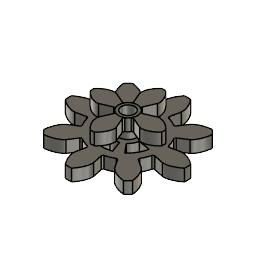
Gear 2 (Autodesk Fusion 360 design; units mm, degrees)
description: Spur Gear; Module: 12.700000; Num Teeth: 8; Pressure Angle: 20.000000; Backlash: 0.00 mm
description: Spur Gear; Module: 12.700000; Num Teeth: 4; Pressure Angle: 20.000000; Backlash: 0.00 mm
Autodesk Fusion 360 part; units mm, degrees
(part 1 of 2)
sketch "Sketch1" plane through (0, 0, 0) normal (0, 0, 1) x (1, 0, 0) in component "Spur Gear (8 teeth)"
  circle A0 centre (0, 0) radius 35.5092
  circle A1 centre (0, 0) radius 6.35
extrude "Extrude1" add sketch "Sketch1" along normal blind 12.7 makes body 1 in component "Spur Gear (8 teeth)"
sketch "Sketch2" plane through (0, 0, 0) normal (0, 0, 1) x (1, 0, 0) in component "Spur Gear (8 teeth)"
  spline S0 degree 5 poles (46.6751, -10.0097) (46.7226, -10.0198) (46.8178, -10.0383) (46.9612, -10.0605) (47.1537, -10.0796) (47.3962, -10.0893) (47.6398, -10.0891) (47.8842, -10.0829) (48.129, -10.0736) (48.374, -10.0619) (48.6191, -10.0476) (48.8645, -10.0296) (49.1102, -10.007) (49.3562, -9.9792) (49.6025, -9.9463) (49.849, -9.9089) (50.0955, -9.8676) (50.3422, -9.8231) (50.5887, -9.7758) (50.8353, -9.7255) (51.0817, -9.6724) (51.3281, -9.6161) (51.5744, -9.5567) (51.8206, -9.4939) (52.0667, -9.428) (52.3127, -9.3591) (52.5584, -9.2873) (52.804, -9.2128) (53.0494, -9.1355) (53.2944, -9.0557) (53.5393, -8.9732) (53.7839, -8.8881) (54.0281, -8.8003) (54.2721, -8.71) (54.5158, -8.617) (54.7591, -8.5215) (55.0021, -8.4236) (55.2447, -8.3232) (55.487, -8.2204) (55.7288, -8.1152) (55.9702, -8.0077) (56.2112, -7.8978) (56.4518, -7.7856) (56.6919, -7.6711) (56.9315, -7.5543) (57.1707, -7.4353) (57.4094, -7.314) (57.6476, -7.1905) (57.8853, -7.0648) (58.1224, -6.937) (58.3591, -6.807) (58.5951, -6.6749) (58.8307, -6.5406) (59.0656, -6.4043) (59.3, -6.2659) (59.5337, -6.1254) (59.7669, -5.9828) (59.9994, -5.8383) (60.2314, -5.6917) (60.4627, -5.5431) (60.6933, -5.3925) (60.9233, -5.24) (61.1526, -5.0855) (61.3813, -4.929) (61.6093, -4.7706) (61.8365, -4.6103) (62.0631, -4.4481) (62.2889, -4.2841) (62.5141, -4.1181) (62.7384, -3.9503) (62.9621, -3.7806) (63.1404, -3.6434) (63.2738, -3.5397) (63.3626, -3.4702) (63.407, -3.4353) knots 0 0 0 0 0 0 0.01428571 0.02857143 0.04285714 0.05714286 0.07142857 0.08571429 0.1 0.11428571 0.12857143 0.14285714 0.15714286 0.17142857 0.18571429 0.2 0.21428571 0.22857143 0.24285714 0.25714286 0.27142857 0.28571429 0.3 0.31428571 0.32857143 0.34285714 0.35714286 0.37142857 0.38571429 0.4 0.41428571 0.42857143 0.44285714 0.45714286 0.47142857 0.48571429 0.5 0.51428571 0.52857143 0.54285714 0.55714286 0.57142857 0.58571429 0.6 0.61428571 0.62857143 0.64285714 0.65714286 0.67142857 0.68571429 0.7 0.71428571 0.72857143 0.74285714 0.75714286 0.77142857 0.78571429 0.8 0.81428571 0.82857143 0.84285714 0.85714286 0.87142857 0.88571429 0.9 0.91428571 0.92857143 0.94285714 0.95714286 0.97142857 0.98571429 1 1 1 1 1 1
  spline S1 degree 5 poles (46.6751, 10.0097) (46.7226, 10.0198) (46.8178, 10.0383) (46.9612, 10.0605) (47.1537, 10.0796) (47.3962, 10.0893) (47.6398, 10.0891) (47.8842, 10.0829) (48.129, 10.0736) (48.374, 10.0619) (48.6191, 10.0476) (48.8645, 10.0296) (49.1102, 10.007) (49.3562, 9.9792) (49.6025, 9.9463) (49.849, 9.9089) (50.0955, 9.8676) (50.3422, 9.8231) (50.5887, 9.7758) (50.8353, 9.7255) (51.0817, 9.6724) (51.3281, 9.6161) (51.5744, 9.5567) (51.8206, 9.4939) (52.0667, 9.428) (52.3127, 9.3591) (52.5584, 9.2873) (52.804, 9.2128) (53.0494, 9.1355) (53.2944, 9.0557) (53.5393, 8.9732) (53.7839, 8.8881) (54.0281, 8.8003) (54.2721, 8.71) (54.5158, 8.617) (54.7591, 8.5215) (55.0021, 8.4236) (55.2447, 8.3232) (55.487, 8.2204) (55.7288, 8.1152) (55.9702, 8.0077) (56.2112, 7.8978) (56.4518, 7.7856) (56.6919, 7.6711) (56.9315, 7.5543) (57.1707, 7.4353) (57.4094, 7.314) (57.6476, 7.1905) (57.8853, 7.0648) (58.1224, 6.937) (58.3591, 6.807) (58.5951, 6.6749) (58.8307, 6.5406) (59.0656, 6.4043) (59.3, 6.2659) (59.5337, 6.1254) (59.7669, 5.9828) (59.9994, 5.8383) (60.2314, 5.6917) (60.4627, 5.5431) (60.6933, 5.3925) (60.9233, 5.24) (61.1526, 5.0855) (61.3813, 4.929) (61.6093, 4.7706) (61.8365, 4.6103) (62.0631, 4.4481) (62.2889, 4.2841) (62.5141, 4.1181) (62.7384, 3.9503) (62.9621, 3.7806) (63.1404, 3.6434) (63.2738, 3.5397) (63.3626, 3.4702) (63.407, 3.4353) knots 0 0 0 0 0 0 0.01428571 0.02857143 0.04285714 0.05714286 0.07142857 0.08571429 0.1 0.11428571 0.12857143 0.14285714 0.15714286 0.17142857 0.18571429 0.2 0.21428571 0.22857143 0.24285714 0.25714286 0.27142857 0.28571429 0.3 0.31428571 0.32857143 0.34285714 0.35714286 0.37142857 0.38571429 0.4 0.41428571 0.42857143 0.44285714 0.45714286 0.47142857 0.48571429 0.5 0.51428571 0.52857143 0.54285714 0.55714286 0.57142857 0.58571429 0.6 0.61428571 0.62857143 0.64285714 0.65714286 0.67142857 0.68571429 0.7 0.71428571 0.72857143 0.74285714 0.75714286 0.77142857 0.78571429 0.8 0.81428571 0.82857143 0.84285714 0.85714286 0.87142857 0.88571429 0.9 0.91428571 0.92857143 0.94285714 0.95714286 0.97142857 0.98571429 1 1 1 1 1 1
  arc A0 (63.407, -3.4353) -> (63.407, 3.4353) centre (0, 0) ccw
  line L0 (34.71, -7.4458) -> (46.6751, -10.0097)
  line L1 (34.71, 7.4458) -> (46.6751, 10.0097)
  line L2 (34.71, -7.4458) -> (34.71, 7.4458)
  point P0 (47.8104, -10.0842)
  point P1 (48.974, -10.0189)
  point P2 (50.155, -9.8564)
  point P3 (51.3487, -9.6105)
  point P4 (52.5517, -9.2886)
  point P5 (53.7613, -8.8954)
  point P6 (54.975, -8.434)
  point P7 (56.1906, -7.9067)
  point P8 (57.4059, -7.3152)
  point P9 (58.6189, -6.6609)
  point P10 (59.8275, -5.9448)
  point P11 (61.0296, -5.168)
  point P12 (62.2235, -4.3313)
  point P13 (47.8104, 10.0842)
  point P14 (48.974, 10.0189)
  point P15 (50.155, 9.8564)
  point P16 (51.3487, 9.6105)
  point P17 (52.5517, 9.2886)
  point P18 (53.7613, 8.8954)
  point P19 (54.975, 8.434)
  point P20 (56.1906, 7.9067)
  point P21 (57.4059, 7.3152)
  point P22 (58.6189, 6.6609)
  point P23 (59.8275, 5.9448)
  point P24 (61.0296, 5.168)
  point P25 (62.2235, 4.3313)
extrude "Extrude2" add sketch "Sketch2" along normal blind 12.7 bodies 1 in component "Spur Gear (8 teeth)"
fillet "Fillet1" radius 1.5875 2 edges at (34.7194, -7.4478, 6.35) (34.7194, 7.4478, 6.35) on bodies 1 in component "Spur Gear (8 teeth)"
pattern_circular "C-Pattern1" count 8 over 360 about axis through (0, 0, 0) along (0, 0, 1) of "Extrude2", "Fillet1" in component "Spur Gear (8 teeth)"
sketch "Sketch3" plane through (0, 0, 0) normal (0, 0, 1) x (1, 0, 0) in component "Spur Gear (8 teeth)"
  circle A0 centre (0, 0) radius 50.8 construction
sketch "Sketch1 (2)" plane through (0, 0, 0) normal (0, 0, 1) x (1, 0, 0) in component "Spur Gear (4 teeth)"
  circle A0 centre (0, 0) radius 10.1092
  circle A1 centre (0, 0) radius 6.35
extrude "Extrude1'" add sketch "Sketch1 (2)" along normal blind 12.7 separate body makes body 2 in component "Spur Gear (4 teeth)"
sketch "Sketch2 (2)" plane through (0, 0, 0) normal (0, 0, 1) x (1, 0, 0) in component "Spur Gear (4 teeth)"
  spline S0 degree 5 poles (21.9128, -9.4616) (21.9552, -9.4799) (22.0407, -9.5141) (22.1712, -9.5583) (22.3491, -9.6037) (22.5768, -9.6426) (22.8081, -9.6692) (23.0414, -9.6889) (23.2758, -9.7048) (23.5109, -9.7174) (23.7467, -9.7262) (23.9837, -9.7295) (24.2219, -9.7262) (24.4615, -9.7158) (24.7023, -9.6987) (24.9439, -9.6758) (25.1862, -9.648) (25.4288, -9.6159) (25.6717, -9.5798) (25.9149, -9.5397) (26.1582, -9.4952) (26.4018, -9.4462) (26.6456, -9.3926) (26.8896, -9.3344) (27.1337, -9.2719) (27.3777, -9.2051) (27.6217, -9.1343) (27.8655, -9.0596) (28.109, -8.9811) (28.3523, -8.8987) (28.5954, -8.8125) (28.838, -8.7225) (29.0803, -8.6286) (29.3222, -8.531) (29.5637, -8.4296) (29.8046, -8.3246) (30.045, -8.216) (30.2848, -8.1038) (30.5239, -7.9882) (30.7623, -7.869) (31.0001, -7.7465) (31.2371, -7.6205) (31.4733, -7.491) (31.7087, -7.3583) (31.9432, -7.2221) (32.1769, -7.0827) (32.4096, -6.9401) (32.6414, -6.7942) (32.8722, -6.6451) (33.1019, -6.4928) (33.3306, -6.3374) (33.5583, -6.1789) (33.7848, -6.0173) (34.0102, -5.8526) (34.2343, -5.6849) (34.4573, -5.5142) (34.6791, -5.3405) (34.8996, -5.1639) (35.1188, -4.9843) (35.3367, -4.8018) (35.5532, -4.6165) (35.7684, -4.4283) (35.9823, -4.2373) (36.1947, -4.0436) (36.4056, -3.847) (36.6151, -3.6477) (36.823, -3.4457) (37.0294, -3.241) (37.2343, -3.0337) (37.4376, -2.8237) (37.6393, -2.6111) (37.7995, -2.4389) (37.9189, -2.3086) (37.9982, -2.2212) (38.0377, -2.1774) knots 0 0 0 0 0 0 0.01428571 0.02857143 0.04285714 0.05714286 0.07142857 0.08571429 0.1 0.11428571 0.12857143 0.14285714 0.15714286 0.17142857 0.18571429 0.2 0.21428571 0.22857143 0.24285714 0.25714286 0.27142857 0.28571429 0.3 0.31428571 0.32857143 0.34285714 0.35714286 0.37142857 0.38571429 0.4 0.41428571 0.42857143 0.44285714 0.45714286 0.47142857 0.48571429 0.5 0.51428571 0.52857143 0.54285714 0.55714286 0.57142857 0.58571429 0.6 0.61428571 0.62857143 0.64285714 0.65714286 0.67142857 0.68571429 0.7 0.71428571 0.72857143 0.74285714 0.75714286 0.77142857 0.78571429 0.8 0.81428571 0.82857143 0.84285714 0.85714286 0.87142857 0.88571429 0.9 0.91428571 0.92857143 0.94285714 0.95714286 0.97142857 0.98571429 1 1 1 1 1 1
  spline S1 degree 5 poles (21.9128, 9.4616) (21.9552, 9.4799) (22.0407, 9.5141) (22.1712, 9.5583) (22.3491, 9.6037) (22.5768, 9.6426) (22.8081, 9.6692) (23.0414, 9.6889) (23.2758, 9.7048) (23.5109, 9.7174) (23.7467, 9.7262) (23.9837, 9.7295) (24.2219, 9.7262) (24.4615, 9.7158) (24.7023, 9.6987) (24.9439, 9.6758) (25.1862, 9.648) (25.4288, 9.6159) (25.6717, 9.5798) (25.9149, 9.5397) (26.1582, 9.4952) (26.4018, 9.4462) (26.6456, 9.3926) (26.8896, 9.3344) (27.1337, 9.2719) (27.3777, 9.2051) (27.6217, 9.1343) (27.8655, 9.0596) (28.109, 8.9811) (28.3523, 8.8987) (28.5954, 8.8125) (28.838, 8.7225) (29.0803, 8.6286) (29.3222, 8.531) (29.5637, 8.4296) (29.8046, 8.3246) (30.045, 8.216) (30.2848, 8.1038) (30.5239, 7.9882) (30.7623, 7.869) (31.0001, 7.7465) (31.2371, 7.6205) (31.4733, 7.491) (31.7087, 7.3583) (31.9432, 7.2221) (32.1769, 7.0827) (32.4096, 6.9401) (32.6414, 6.7942) (32.8722, 6.6451) (33.1019, 6.4928) (33.3306, 6.3374) (33.5583, 6.1789) (33.7848, 6.0173) (34.0102, 5.8526) (34.2343, 5.6849) (34.4573, 5.5142) (34.6791, 5.3405) (34.8996, 5.1639) (35.1188, 4.9843) (35.3367, 4.8018) (35.5532, 4.6165) (35.7684, 4.4283) (35.9823, 4.2373) (36.1947, 4.0436) (36.4056, 3.847) (36.6151, 3.6477) (36.823, 3.4457) (37.0294, 3.241) (37.2343, 3.0337) (37.4376, 2.8237) (37.6393, 2.6111) (37.7995, 2.4389) (37.9189, 2.3086) (37.9982, 2.2212) (38.0377, 2.1774) knots 0 0 0 0 0 0 0.01428571 0.02857143 0.04285714 0.05714286 0.07142857 0.08571429 0.1 0.11428571 0.12857143 0.14285714 0.15714286 0.17142857 0.18571429 0.2 0.21428571 0.22857143 0.24285714 0.25714286 0.27142857 0.28571429 0.3 0.31428571 0.32857143 0.34285714 0.35714286 0.37142857 0.38571429 0.4 0.41428571 0.42857143 0.44285714 0.45714286 0.47142857 0.48571429 0.5 0.51428571 0.52857143 0.54285714 0.55714286 0.57142857 0.58571429 0.6 0.61428571 0.62857143 0.64285714 0.65714286 0.67142857 0.68571429 0.7 0.71428571 0.72857143 0.74285714 0.75714286 0.77142857 0.78571429 0.8 0.81428571 0.82857143 0.84285714 0.85714286 0.87142857 0.88571429 0.9 0.91428571 0.92857143 0.94285714 0.95714286 0.97142857 0.98571429 1 1 1 1 1 1
  arc A0 (38.0377, -2.1774) -> (38.0377, 2.1774) centre (0, 0) ccw
  line L0 (9.2718, -4.0074) -> (21.9128, -9.4616)
  line L1 (9.2718, 4.0074) -> (21.9128, 9.4616)
  line L2 (9.2718, -4.0074) -> (9.2718, 4.0074)
  point P0 (22.9255, -9.6784)
  point P1 (24.0052, -9.7278)
  point P2 (25.1271, -9.6541)
  point P3 (26.2802, -9.4701)
  point P4 (27.4564, -9.1817)
  point P5 (28.6488, -8.792)
  point P6 (29.8509, -8.303)
  point P7 (31.0565, -7.7159)
  point P8 (32.2598, -7.0314)
  point P9 (33.4549, -6.2504)
  point P10 (34.636, -5.3736)
  point P11 (35.7973, -4.4018)
  point P12 (36.9331, -3.336)
  point P13 (22.9255, 9.6784)
  point P14 (24.0052, 9.7278)
  point P15 (25.1271, 9.6541)
  point P16 (26.2802, 9.4701)
  point P17 (27.4564, 9.1817)
  point P18 (28.6488, 8.792)
  point P19 (29.8509, 8.303)
  point P20 (31.0565, 7.7159)
  point P21 (32.2598, 7.0314)
  point P22 (33.4549, 6.2504)
  point P23 (34.636, 5.3736)
  point P24 (35.7973, 4.4018)
  point P25 (36.9331, 3.336)
extrude "Extrude2'" add sketch "Sketch2 (2)" along normal blind 12.7 bodies 2 in component "Spur Gear (4 teeth)"
fillet "Fillet1'" radius 1.5875 2 edges at (9.2795, -4.0107, 6.35) (9.2795, 4.0107, 6.35) on bodies 2 in component "Spur Gear (4 teeth)"
pattern_circular "C-Pattern1'" count 4 over 360 about axis through (0, 0, 0) along (0, 0, 1) of "Extrude2'", "Fillet1'" in component "Spur Gear (4 teeth)"
sketch "Sketch3 (2)" plane through (0, 0, 0) normal (0, 0, 1) x (1, 0, 0) in component "Spur Gear (4 teeth)"
  circle A0 centre (0, 0) radius 25.4 construction
move_body "Move1" bodies 2 to x (1, 0, 0) y (0, 1, 0) z (0, 0, 1) at (0, 0, 20) in component "Spur Gear (4 teeth)"
sketch "Sketch1 (3)" plane through (0, 0, 0) normal (0, 0, -1) x (1, 0, 0)
  circle A0 centre (0, 0) radius 6.35
  arc A1 (7.7732, 36.2381) -> (8.9264, 34.3689) centre (9.3255, 35.9054) ccw
  line L0 (7.7732, 36.2381) -> (10.0097, 46.6751)
  spline S0 degree 5 poles (10.0097, 46.6751) (10.0198, 46.7226) (10.0383, 46.8178) (10.0605, 46.9612) (10.0796, 47.1537) (10.0893, 47.3962) (10.0891, 47.6398) (10.0829, 47.8842) (10.0736, 48.129) (10.0619, 48.374) (10.0476, 48.6191) (10.0296, 48.8645) (10.007, 49.1102) (9.9792, 49.3562) (9.9463, 49.6025) (9.9089, 49.849) (9.8676, 50.0955) (9.8231, 50.3422) (9.7758, 50.5887) (9.7255, 50.8353) (9.6724, 51.0817) (9.6161, 51.3281) (9.5567, 51.5744) (9.4939, 51.8206) (9.428, 52.0667) (9.3591, 52.3127) (9.2873, 52.5584) (9.2128, 52.804) (9.1355, 53.0494) (9.0557, 53.2944) (8.9732, 53.5393) (8.8881, 53.7839) (8.8003, 54.0281) (8.71, 54.2721) (8.617, 54.5158) (8.5215, 54.7591) (8.4236, 55.0021) (8.3232, 55.2447) (8.2204, 55.487) (8.1152, 55.7288) (8.0077, 55.9702) (7.8978, 56.2112) (7.7856, 56.4518) (7.6711, 56.6919) (7.5543, 56.9315) (7.4353, 57.1707) (7.314, 57.4094) (7.1905, 57.6476) (7.0648, 57.8853) (6.937, 58.1224) (6.807, 58.3591) (6.6749, 58.5951) (6.5406, 58.8307) (6.4043, 59.0656) (6.2659, 59.3) (6.1254, 59.5337) (5.9828, 59.7669) (5.8383, 59.9994) (5.6917, 60.2314) (5.5431, 60.4627) (5.3925, 60.6933) (5.24, 60.9233) (5.0855, 61.1526) (4.929, 61.3813) (4.7706, 61.6093) (4.6103, 61.8365) (4.4481, 62.0631) (4.2841, 62.2889) (4.1181, 62.5141) (3.9503, 62.7384) (3.7806, 62.9621) (3.6434, 63.1404) (3.5397, 63.2738) (3.4702, 63.3626) (3.4353, 63.407) knots 0 0 0 0 0 0 0.01428571 0.02857143 0.04285714 0.05714286 0.07142857 0.08571429 0.1 0.11428571 0.12857143 0.14285714 0.15714286 0.17142857 0.18571429 0.2 0.21428571 0.22857143 0.24285714 0.25714286 0.27142857 0.28571429 0.3 0.31428571 0.32857143 0.34285714 0.35714286 0.37142857 0.38571429 0.4 0.41428571 0.42857143 0.44285714 0.45714286 0.47142857 0.48571429 0.5 0.51428571 0.52857143 0.54285714 0.55714286 0.57142857 0.58571429 0.6 0.61428571 0.62857143 0.64285714 0.65714286 0.67142857 0.68571429 0.7 0.71428571 0.72857143 0.74285714 0.75714286 0.77142857 0.78571429 0.8 0.81428571 0.82857143 0.84285714 0.85714286 0.87142857 0.88571429 0.9 0.91428571 0.92857143 0.94285714 0.95714286 0.97142857 0.98571429 1 1 1 1 1 1
  arc A2 (3.4353, 63.407) -> (-3.4353, 63.407) centre (0, 0) ccw
  spline S1 degree 5 poles (-10.0097, 46.6751) (-10.0198, 46.7226) (-10.0383, 46.8178) (-10.0605, 46.9612) (-10.0796, 47.1537) (-10.0893, 47.3962) (-10.0891, 47.6398) (-10.0829, 47.8842) (-10.0736, 48.129) (-10.0619, 48.374) (-10.0476, 48.6191) (-10.0296, 48.8645) (-10.007, 49.1102) (-9.9792, 49.3562) (-9.9463, 49.6025) (-9.9089, 49.849) (-9.8676, 50.0955) (-9.8231, 50.3422) (-9.7758, 50.5887) (-9.7255, 50.8353) (-9.6724, 51.0817) (-9.6161, 51.3281) (-9.5567, 51.5744) (-9.4939, 51.8206) (-9.428, 52.0667) (-9.3591, 52.3127) (-9.2873, 52.5584) (-9.2128, 52.804) (-9.1355, 53.0494) (-9.0557, 53.2944) (-8.9732, 53.5393) (-8.8881, 53.7839) (-8.8003, 54.0281) (-8.71, 54.2721) (-8.617, 54.5158) (-8.5215, 54.7591) (-8.4236, 55.0021) (-8.3232, 55.2447) (-8.2204, 55.487) (-8.1152, 55.7288) (-8.0077, 55.9702) (-7.8978, 56.2112) (-7.7856, 56.4518) (-7.6711, 56.6919) (-7.5543, 56.9315) (-7.4353, 57.1707) (-7.314, 57.4094) (-7.1905, 57.6476) (-7.0648, 57.8853) (-6.937, 58.1224) (-6.807, 58.3591) (-6.6749, 58.5951) (-6.5406, 58.8307) (-6.4043, 59.0656) (-6.2659, 59.3) (-6.1254, 59.5337) (-5.9828, 59.7669) (-5.8383, 59.9994) (-5.6917, 60.2314) (-5.5431, 60.4627) (-5.3925, 60.6933) (-5.24, 60.9233) (-5.0855, 61.1526) (-4.929, 61.3813) (-4.7706, 61.6093) (-4.6103, 61.8365) (-4.4481, 62.0631) (-4.2841, 62.2889) (-4.1181, 62.5141) (-3.9503, 62.7384) (-3.7806, 62.9621) (-3.6434, 63.1404) (-3.5397, 63.2738) (-3.4702, 63.3626) (-3.4353, 63.407) knots 0 0 0 0 0 0 0.01428571 0.02857143 0.04285714 0.05714286 0.07142857 0.08571429 0.1 0.11428571 0.12857143 0.14285714 0.15714286 0.17142857 0.18571429 0.2 0.21428571 0.22857143 0.24285714 0.25714286 0.27142857 0.28571429 0.3 0.31428571 0.32857143 0.34285714 0.35714286 0.37142857 0.38571429 0.4 0.41428571 0.42857143 0.44285714 0.45714286 0.47142857 0.48571429 0.5 0.51428571 0.52857143 0.54285714 0.55714286 0.57142857 0.58571429 0.6 0.61428571 0.62857143 0.64285714 0.65714286 0.67142857 0.68571429 0.7 0.71428571 0.72857143 0.74285714 0.75714286 0.77142857 0.78571429 0.8 0.81428571 0.82857143 0.84285714 0.85714286 0.87142857 0.88571429 0.9 0.91428571 0.92857143 0.94285714 0.95714286 0.97142857 0.98571429 1 1 1 1 1 1
  line L1 (-10.0097, 46.6751) -> (-7.7732, 36.2381)
  arc A3 (-8.9264, 34.3689) -> (-7.7732, 36.2381) centre (-9.3255, 35.9054) ccw
  arc A4 (-8.9264, 34.3689) -> (-17.9906, 30.6144) centre (0, 0) ccw
  arc A5 (-20.1277, 31.1207) -> (-17.9906, 30.6144) centre (-18.7949, 31.9831) ccw
  line L2 (-20.1277, 31.1207) -> (-25.9264, 40.0822)
  spline S2 degree 5 poles (-25.9264, 40.0822) (-25.9528, 40.123) (-26.007, 40.2033) (-26.0927, 40.3204) (-26.2154, 40.4701) (-26.3799, 40.6484) (-26.5524, 40.8205) (-26.7296, 40.989) (-26.9092, 41.1554) (-27.0907, 41.3204) (-27.2742, 41.4836) (-27.4604, 41.6444) (-27.6501, 41.8022) (-27.8437, 41.9565) (-28.0411, 42.1074) (-28.2419, 42.2552) (-28.4454, 42.4004) (-28.6513, 42.5433) (-28.8591, 42.6841) (-29.069, 42.823) (-29.2808, 42.9596) (-29.4948, 43.0941) (-29.711, 43.2262) (-29.9295, 43.3559) (-30.1501, 43.4833) (-30.3728, 43.6085) (-30.5973, 43.7315) (-30.8237, 43.8525) (-31.0517, 43.9714) (-31.2815, 44.0882) (-31.513, 44.203) (-31.7461, 44.3158) (-31.9809, 44.4264) (-32.2173, 44.5351) (-32.4553, 44.6416) (-32.6949, 44.7462) (-32.936, 44.8487) (-33.1785, 44.9493) (-33.4225, 45.0479) (-33.6679, 45.1445) (-33.9146, 45.2392) (-34.1627, 45.3319) (-34.4122, 45.4227) (-34.6629, 45.5115) (-34.915, 45.5984) (-35.1683, 45.6833) (-35.4228, 45.7664) (-35.6786, 45.8475) (-35.9355, 45.9267) (-36.1936, 46.004) (-36.4528, 46.0794) (-36.7132, 46.1529) (-36.9746, 46.2245) (-37.2372, 46.2942) (-37.5008, 46.362) (-37.7654, 46.428) (-38.0311, 46.4921) (-38.2977, 46.5543) (-38.5654, 46.6146) (-38.834, 46.6731) (-39.1036, 46.7297) (-39.3741, 46.7845) (-39.6455, 46.8374) (-39.9178, 46.8885) (-40.191, 46.9377) (-40.465, 46.985) (-40.7399, 47.0305) (-41.0156, 47.0742) (-41.2922, 47.1161) (-41.5695, 47.1561) (-41.8476, 47.1942) (-42.0707, 47.2233) (-42.2384, 47.2443) (-42.3504, 47.2579) (-42.4064, 47.2647) knots 0 0 0 0 0 0 0.01428571 0.02857143 0.04285714 0.05714286 0.07142857 0.08571429 0.1 0.11428571 0.12857143 0.14285714 0.15714286 0.17142857 0.18571429 0.2 0.21428571 0.22857143 0.24285714 0.25714286 0.27142857 0.28571429 0.3 0.31428571 0.32857143 0.34285714 0.35714286 0.37142857 0.38571429 0.4 0.41428571 0.42857143 0.44285714 0.45714286 0.47142857 0.48571429 0.5 0.51428571 0.52857143 0.54285714 0.55714286 0.57142857 0.58571429 0.6 0.61428571 0.62857143 0.64285714 0.65714286 0.67142857 0.68571429 0.7 0.71428571 0.72857143 0.74285714 0.75714286 0.77142857 0.78571429 0.8 0.81428571 0.82857143 0.84285714 0.85714286 0.87142857 0.88571429 0.9 0.91428571 0.92857143 0.94285714 0.95714286 0.97142857 0.98571429 1 1 1 1 1 1
  arc A6 (-42.4064, 47.2647) -> (-47.2647, 42.4064) centre (0, 0) ccw
  spline S3 degree 5 poles (-40.0822, 25.9264) (-40.123, 25.9528) (-40.2033, 26.007) (-40.3204, 26.0927) (-40.4701, 26.2154) (-40.6484, 26.3799) (-40.8205, 26.5524) (-40.989, 26.7296) (-41.1554, 26.9092) (-41.3204, 27.0907) (-41.4836, 27.2742) (-41.6444, 27.4604) (-41.8022, 27.6501) (-41.9565, 27.8437) (-42.1074, 28.0411) (-42.2552, 28.2419) (-42.4004, 28.4454) (-42.5433, 28.6513) (-42.6841, 28.8591) (-42.823, 29.069) (-42.9596, 29.2808) (-43.0941, 29.4948) (-43.2262, 29.711) (-43.3559, 29.9295) (-43.4833, 30.1501) (-43.6085, 30.3728) (-43.7315, 30.5973) (-43.8525, 30.8237) (-43.9714, 31.0517) (-44.0882, 31.2815) (-44.203, 31.513) (-44.3158, 31.7461) (-44.4264, 31.9809) (-44.5351, 32.2173) (-44.6416, 32.4553) (-44.7462, 32.6949) (-44.8487, 32.936) (-44.9493, 33.1785) (-45.0479, 33.4225) (-45.1445, 33.6679) (-45.2392, 33.9146) (-45.3319, 34.1627) (-45.4227, 34.4122) (-45.5115, 34.6629) (-45.5984, 34.915) (-45.6833, 35.1683) (-45.7664, 35.4228) (-45.8475, 35.6786) (-45.9267, 35.9355) (-46.004, 36.1936) (-46.0794, 36.4528) (-46.1529, 36.7132) (-46.2245, 36.9746) (-46.2942, 37.2372) (-46.362, 37.5008) (-46.428, 37.7654) (-46.4921, 38.0311) (-46.5543, 38.2977) (-46.6146, 38.5654) (-46.6731, 38.834) (-46.7297, 39.1036) (-46.7845, 39.3741) (-46.8374, 39.6455) (-46.8885, 39.9178) (-46.9377, 40.191) (-46.985, 40.465) (-47.0305, 40.7399) (-47.0742, 41.0156) (-47.1161, 41.2922) (-47.1561, 41.5695) (-47.1942, 41.8476) (-47.2233, 42.0707) (-47.2443, 42.2384) (-47.2579, 42.3504) (-47.2647, 42.4064) knots 0 0 0 0 0 0 0.01428571 0.02857143 0.04285714 0.05714286 0.07142857 0.08571429 0.1 0.11428571 0.12857143 0.14285714 0.15714286 0.17142857 0.18571429 0.2 0.21428571 0.22857143 0.24285714 0.25714286 0.27142857 0.28571429 0.3 0.31428571 0.32857143 0.34285714 0.35714286 0.37142857 0.38571429 0.4 0.41428571 0.42857143 0.44285714 0.45714286 0.47142857 0.48571429 0.5 0.51428571 0.52857143 0.54285714 0.55714286 0.57142857 0.58571429 0.6 0.61428571 0.62857143 0.64285714 0.65714286 0.67142857 0.68571429 0.7 0.71428571 0.72857143 0.74285714 0.75714286 0.77142857 0.78571429 0.8 0.81428571 0.82857143 0.84285714 0.85714286 0.87142857 0.88571429 0.9 0.91428571 0.92857143 0.94285714 0.95714286 0.97142857 0.98571429 1 1 1 1 1 1
  line L3 (-40.0822, 25.9264) -> (-31.1207, 20.1277)
  arc A7 (-30.6144, 17.9906) -> (-31.1207, 20.1277) centre (-31.9831, 18.7949) ccw
  arc A8 (-30.6144, 17.9906) -> (-34.3689, 8.9264) centre (0, 0) ccw
  arc A9 (-36.2381, 7.7732) -> (-34.3689, 8.9264) centre (-35.9054, 9.3255) ccw
  line L4 (-36.2381, 7.7732) -> (-46.6751, 10.0097)
  spline S4 degree 5 poles (-46.6751, 10.0097) (-46.7226, 10.0198) (-46.8178, 10.0383) (-46.9612, 10.0605) (-47.1537, 10.0796) (-47.3962, 10.0893) (-47.6398, 10.0891) (-47.8842, 10.0829) (-48.129, 10.0736) (-48.374, 10.0619) (-48.6191, 10.0476) (-48.8645, 10.0296) (-49.1102, 10.007) (-49.3562, 9.9792) (-49.6025, 9.9463) (-49.849, 9.9089) (-50.0955, 9.8676) (-50.3422, 9.8231) (-50.5887, 9.7758) (-50.8353, 9.7255) (-51.0817, 9.6724) (-51.3281, 9.6161) (-51.5744, 9.5567) (-51.8206, 9.4939) (-52.0667, 9.428) (-52.3127, 9.3591) (-52.5584, 9.2873) (-52.804, 9.2128) (-53.0494, 9.1355) (-53.2944, 9.0557) (-53.5393, 8.9732) (-53.7839, 8.8881) (-54.0281, 8.8003) (-54.2721, 8.71) (-54.5158, 8.617) (-54.7591, 8.5215) (-55.0021, 8.4236) (-55.2447, 8.3232) (-55.487, 8.2204) (-55.7288, 8.1152) (-55.9702, 8.0077) (-56.2112, 7.8978) (-56.4518, 7.7856) (-56.6919, 7.6711) (-56.9315, 7.5543) (-57.1707, 7.4353) (-57.4094, 7.314) (-57.6476, 7.1905) (-57.8853, 7.0648) (-58.1224, 6.937) (-58.3591, 6.807) (-58.5951, 6.6749) (-58.8307, 6.5406) (-59.0656, 6.4043) (-59.3, 6.2659) (-59.5337, 6.1254) (-59.7669, 5.9828) (-59.9994, 5.8383) (-60.2314, 5.6917) (-60.4627, 5.5431) (-60.6933, 5.3925) (-60.9233, 5.24) (-61.1526, 5.0855) (-61.3813, 4.929) (-61.6093, 4.7706) (-61.8365, 4.6103) (-62.0631, 4.4481) (-62.2889, 4.2841) (-62.5141, 4.1181) (-62.7384, 3.9503) (-62.9621, 3.7806) (-63.1404, 3.6434) (-63.2738, 3.5397) (-63.3626, 3.4702) (-63.407, 3.4353) knots 0 0 0 0 0 0 0.01428571 0.02857143 0.04285714 0.05714286 0.07142857 0.08571429 0.1 0.11428571 0.12857143 0.14285714 0.15714286 0.17142857 0.18571429 0.2 0.21428571 0.22857143 0.24285714 0.25714286 0.27142857 0.28571429 0.3 0.31428571 0.32857143 0.34285714 0.35714286 0.37142857 0.38571429 0.4 0.41428571 0.42857143 0.44285714 0.45714286 0.47142857 0.48571429 0.5 0.51428571 0.52857143 0.54285714 0.55714286 0.57142857 0.58571429 0.6 0.61428571 0.62857143 0.64285714 0.65714286 0.67142857 0.68571429 0.7 0.71428571 0.72857143 0.74285714 0.75714286 0.77142857 0.78571429 0.8 0.81428571 0.82857143 0.84285714 0.85714286 0.87142857 0.88571429 0.9 0.91428571 0.92857143 0.94285714 0.95714286 0.97142857 0.98571429 1 1 1 1 1 1
  arc A10 (-63.407, 3.4353) -> (-63.407, -3.4353) centre (0, 0) ccw
  spline S5 degree 5 poles (-46.6751, -10.0097) (-46.7226, -10.0198) (-46.8178, -10.0383) (-46.9612, -10.0605) (-47.1537, -10.0796) (-47.3962, -10.0893) (-47.6398, -10.0891) (-47.8842, -10.0829) (-48.129, -10.0736) (-48.374, -10.0619) (-48.6191, -10.0476) (-48.8645, -10.0296) (-49.1102, -10.007) (-49.3562, -9.9792) (-49.6025, -9.9463) (-49.849, -9.9089) (-50.0955, -9.8676) (-50.3422, -9.8231) (-50.5887, -9.7758) (-50.8353, -9.7255) (-51.0817, -9.6724) (-51.3281, -9.6161) (-51.5744, -9.5567) (-51.8206, -9.4939) (-52.0667, -9.428) (-52.3127, -9.3591) (-52.5584, -9.2873) (-52.804, -9.2128) (-53.0494, -9.1355) (-53.2944, -9.0557) (-53.5393, -8.9732) (-53.7839, -8.8881) (-54.0281, -8.8003) (-54.2721, -8.71) (-54.5158, -8.617) (-54.7591, -8.5215) (-55.0021, -8.4236) (-55.2447, -8.3232) (-55.487, -8.2204) (-55.7288, -8.1152) (-55.9702, -8.0077) (-56.2112, -7.8978) (-56.4518, -7.7856) (-56.6919, -7.6711) (-56.9315, -7.5543) (-57.1707, -7.4353) (-57.4094, -7.314) (-57.6476, -7.1905) (-57.8853, -7.0648) (-58.1224, -6.937) (-58.3591, -6.807) (-58.5951, -6.6749) (-58.8307, -6.5406) (-59.0656, -6.4043) (-59.3, -6.2659) (-59.5337, -6.1254) (-59.7669, -5.9828) (-59.9994, -5.8383) (-60.2314, -5.6917) (-60.4627, -5.5431) (-60.6933, -5.3925) (-60.9233, -5.24) (-61.1526, -5.0855) (-61.3813, -4.929) (-61.6093, -4.7706) (-61.8365, -4.6103) (-62.0631, -4.4481) (-62.2889, -4.2841) (-62.5141, -4.1181) (-62.7384, -3.9503) (-62.9621, -3.7806) (-63.1404, -3.6434) (-63.2738, -3.5397) (-63.3626, -3.4702) (-63.407, -3.4353) knots 0 0 0 0 0 0 0.01428571 0.02857143 0.04285714 0.05714286 0.07142857 0.08571429 0.1 0.11428571 0.12857143 0.14285714 0.15714286 0.17142857 0.18571429 0.2 0.21428571 0.22857143 0.24285714 0.25714286 0.27142857 0.28571429 0.3 0.31428571 0.32857143 0.34285714 0.35714286 0.37142857 0.38571429 0.4 0.41428571 0.42857143 0.44285714 0.45714286 0.47142857 0.48571429 0.5 0.51428571 0.52857143 0.54285714 0.55714286 0.57142857 0.58571429 0.6 0.61428571 0.62857143 0.64285714 0.65714286 0.67142857 0.68571429 0.7 0.71428571 0.72857143 0.74285714 0.75714286 0.77142857 0.78571429 0.8 0.81428571 0.82857143 0.84285714 0.85714286 0.87142857 0.88571429 0.9 0.91428571 0.92857143 0.94285714 0.95714286 0.97142857 0.98571429 1 1 1 1 1 1
  line L5 (-46.6751, -10.0097) -> (-36.2381, -7.7732)
  arc A11 (-34.3689, -8.9264) -> (-36.2381, -7.7732) centre (-35.9054, -9.3255) ccw
  arc A12 (-34.3689, -8.9264) -> (-30.6144, -17.9906) centre (0, 0) ccw
  arc A13 (-31.1207, -20.1277) -> (-30.6144, -17.9906) centre (-31.9831, -18.7949) ccw
  line L6 (-31.1207, -20.1277) -> (-40.0822, -25.9264)
  spline S6 degree 5 poles (-40.0822, -25.9264) (-40.123, -25.9528) (-40.2033, -26.007) (-40.3204, -26.0927) (-40.4701, -26.2154) (-40.6484, -26.3799) (-40.8205, -26.5524) (-40.989, -26.7296) (-41.1554, -26.9092) (-41.3204, -27.0907) (-41.4836, -27.2742) (-41.6444, -27.4604) (-41.8022, -27.6501) (-41.9565, -27.8437) (-42.1074, -28.0411) (-42.2552, -28.2419) (-42.4004, -28.4454) (-42.5433, -28.6513) (-42.6841, -28.8591) (-42.823, -29.069) (-42.9596, -29.2808) (-43.0941, -29.4948) (-43.2262, -29.711) (-43.3559, -29.9295) (-43.4833, -30.1501) (-43.6085, -30.3728) (-43.7315, -30.5973) (-43.8525, -30.8237) (-43.9714, -31.0517) (-44.0882, -31.2815) (-44.203, -31.513) (-44.3158, -31.7461) (-44.4264, -31.9809) (-44.5351, -32.2173) (-44.6416, -32.4553) (-44.7462, -32.6949) (-44.8487, -32.936) (-44.9493, -33.1785) (-45.0479, -33.4225) (-45.1445, -33.6679) (-45.2392, -33.9146) (-45.3319, -34.1627) (-45.4227, -34.4122) (-45.5115, -34.6629) (-45.5984, -34.915) (-45.6833, -35.1683) (-45.7664, -35.4228) (-45.8475, -35.6786) (-45.9267, -35.9355) (-46.004, -36.1936) (-46.0794, -36.4528) (-46.1529, -36.7132) (-46.2245, -36.9746) (-46.2942, -37.2372) (-46.362, -37.5008) (-46.428, -37.7654) (-46.4921, -38.0311) (-46.5543, -38.2977) (-46.6146, -38.5654) (-46.6731, -38.834) (-46.7297, -39.1036) (-46.7845, -39.3741) (-46.8374, -39.6455) (-46.8885, -39.9178) (-46.9377, -40.191) (-46.985, -40.465) (-47.0305, -40.7399) (-47.0742, -41.0156) (-47.1161, -41.2922) (-47.1561, -41.5695) (-47.1942, -41.8476) (-47.2233, -42.0707) (-47.2443, -42.2384) (-47.2579, -42.3504) (-47.2647, -42.4064) knots 0 0 0 0 0 0 0.01428571 0.02857143 0.04285714 0.05714286 0.07142857 0.08571429 0.1 0.11428571 0.12857143 0.14285714 0.15714286 0.17142857 0.18571429 0.2 0.21428571 0.22857143 0.24285714 0.25714286 0.27142857 0.28571429 0.3 0.31428571 0.32857143 0.34285714 0.35714286 0.37142857 0.38571429 0.4 0.41428571 0.42857143 0.44285714 0.45714286 0.47142857 0.48571429 0.5 0.51428571 0.52857143 0.54285714 0.55714286 0.57142857 0.58571429 0.6 0.61428571 0.62857143 0.64285714 0.65714286 0.67142857 0.68571429 0.7 0.71428571 0.72857143 0.74285714 0.75714286 0.77142857 0.78571429 0.8 0.81428571 0.82857143 0.84285714 0.85714286 0.87142857 0.88571429 0.9 0.91428571 0.92857143 0.94285714 0.95714286 0.97142857 0.98571429 1 1 1 1 1 1
  arc A14 (-47.2647, -42.4064) -> (-42.4064, -47.2647) centre (0, 0) ccw
  spline S7 degree 5 poles (-25.9264, -40.0822) (-25.9528, -40.123) (-26.007, -40.2033) (-26.0927, -40.3204) (-26.2154, -40.4701) (-26.3799, -40.6484) (-26.5524, -40.8205) (-26.7296, -40.989) (-26.9092, -41.1554) (-27.0907, -41.3204) (-27.2742, -41.4836) (-27.4604, -41.6444) (-27.6501, -41.8022) (-27.8437, -41.9565) (-28.0411, -42.1074) (-28.2419, -42.2552) (-28.4454, -42.4004) (-28.6513, -42.5433) (-28.8591, -42.6841) (-29.069, -42.823) (-29.2808, -42.9596) (-29.4948, -43.0941) (-29.711, -43.2262) (-29.9295, -43.3559) (-30.1501, -43.4833) (-30.3728, -43.6085) (-30.5973, -43.7315) (-30.8237, -43.8525) (-31.0517, -43.9714) (-31.2815, -44.0882) (-31.513, -44.203) (-31.7461, -44.3158) (-31.9809, -44.4264) (-32.2173, -44.5351) (-32.4553, -44.6416) (-32.6949, -44.7462) (-32.936, -44.8487) (-33.1785, -44.9493) (-33.4225, -45.0479) (-33.6679, -45.1445) (-33.9146, -45.2392) (-34.1627, -45.3319) (-34.4122, -45.4227) (-34.6629, -45.5115) (-34.915, -45.5984) (-35.1683, -45.6833) (-35.4228, -45.7664) (-35.6786, -45.8475) (-35.9355, -45.9267) (-36.1936, -46.004) (-36.4528, -46.0794) (-36.7132, -46.1529) (-36.9746, -46.2245) (-37.2372, -46.2942) (-37.5008, -46.362) (-37.7654, -46.428) (-38.0311, -46.4921) (-38.2977, -46.5543) (-38.5654, -46.6146) (-38.834, -46.6731) (-39.1036, -46.7297) (-39.3741, -46.7845) (-39.6455, -46.8374) (-39.9178, -46.8885) (-40.191, -46.9377) (-40.465, -46.985) (-40.7399, -47.0305) (-41.0156, -47.0742) (-41.2922, -47.1161) (-41.5695, -47.1561) (-41.8476, -47.1942) (-42.0707, -47.2233) (-42.2384, -47.2443) (-42.3504, -47.2579) (-42.4064, -47.2647) knots 0 0 0 0 0 0 0.01428571 0.02857143 0.04285714 0.05714286 0.07142857 0.08571429 0.1 0.11428571 0.12857143 0.14285714 0.15714286 0.17142857 0.18571429 0.2 0.21428571 0.22857143 0.24285714 0.25714286 0.27142857 0.28571429 0.3 0.31428571 0.32857143 0.34285714 0.35714286 0.37142857 0.38571429 0.4 0.41428571 0.42857143 0.44285714 0.45714286 0.47142857 0.48571429 0.5 0.51428571 0.52857143 0.54285714 0.55714286 0.57142857 0.58571429 0.6 0.61428571 0.62857143 0.64285714 0.65714286 0.67142857 0.68571429 0.7 0.71428571 0.72857143 0.74285714 0.75714286 0.77142857 0.78571429 0.8 0.81428571 0.82857143 0.84285714 0.85714286 0.87142857 0.88571429 0.9 0.91428571 0.92857143 0.94285714 0.95714286 0.97142857 0.98571429 1 1 1 1 1 1
  line L7 (-25.9264, -40.0822) -> (-20.1277, -31.1207)
  arc A15 (-17.9906, -30.6144) -> (-20.1277, -31.1207) centre (-18.7949, -31.9831) ccw
  arc A16 (-17.9906, -30.6144) -> (-8.9264, -34.3689) centre (0, 0) ccw
  arc A17 (-7.7732, -36.2381) -> (-8.9264, -34.3689) centre (-9.3255, -35.9054) ccw
  line L8 (-7.7732, -36.2381) -> (-10.0097, -46.6751)
  spline S8 degree 5 poles (-10.0097, -46.6751) (-10.0198, -46.7226) (-10.0383, -46.8178) (-10.0605, -46.9612) (-10.0796, -47.1537) (-10.0893, -47.3962) (-10.0891, -47.6398) (-10.0829, -47.8842) (-10.0736, -48.129) (-10.0619, -48.374) (-10.0476, -48.6191) (-10.0296, -48.8645) (-10.007, -49.1102) (-9.9792, -49.3562) (-9.9463, -49.6025) (-9.9089, -49.849) (-9.8676, -50.0955) (-9.8231, -50.3422) (-9.7758, -50.5887) (-9.7255, -50.8353) (-9.6724, -51.0817) (-9.6161, -51.3281) (-9.5567, -51.5744) (-9.4939, -51.8206) (-9.428, -52.0667) (-9.3591, -52.3127) (-9.2873, -52.5584) (-9.2128, -52.804) (-9.1355, -53.0494) (-9.0557, -53.2944) (-8.9732, -53.5393) (-8.8881, -53.7839) (-8.8003, -54.0281) (-8.71, -54.2721) (-8.617, -54.5158) (-8.5215, -54.7591) (-8.4236, -55.0021) (-8.3232, -55.2447) (-8.2204, -55.487) (-8.1152, -55.7288) (-8.0077, -55.9702) (-7.8978, -56.2112) (-7.7856, -56.4518) (-7.6711, -56.6919) (-7.5543, -56.9315) (-7.4353, -57.1707) (-7.314, -57.4094) (-7.1905, -57.6476) (-7.0648, -57.8853) (-6.937, -58.1224) (-6.807, -58.3591) (-6.6749, -58.5951) (-6.5406, -58.8307) (-6.4043, -59.0656) (-6.2659, -59.3) (-6.1254, -59.5337) (-5.9828, -59.7669) (-5.8383, -59.9994) (-5.6917, -60.2314) (-5.5431, -60.4627) (-5.3925, -60.6933) (-5.24, -60.9233) (-5.0855, -61.1526) (-4.929, -61.3813) (-4.7706, -61.6093) (-4.6103, -61.8365) (-4.4481, -62.0631) (-4.2841, -62.2889) (-4.1181, -62.5141) (-3.9503, -62.7384) (-3.7806, -62.9621) (-3.6434, -63.1404) (-3.5397, -63.2738) (-3.4702, -63.3626) (-3.4353, -63.407) knots 0 0 0 0 0 0 0.01428571 0.02857143 0.04285714 0.05714286 0.07142857 0.08571429 0.1 0.11428571 0.12857143 0.14285714 0.15714286 0.17142857 0.18571429 0.2 0.21428571 0.22857143 0.24285714 0.25714286 0.27142857 0.28571429 0.3 0.31428571 0.32857143 0.34285714 0.35714286 0.37142857 0.38571429 0.4 0.41428571 0.42857143 0.44285714 0.45714286 0.47142857 0.48571429 0.5 0.51428571 0.52857143 0.54285714 0.55714286 0.57142857 0.58571429 0.6 0.61428571 0.62857143 0.64285714 0.65714286 0.67142857 0.68571429 0.7 0.71428571 0.72857143 0.74285714 0.75714286 0.77142857 0.78571429 0.8 0.81428571 0.82857143 0.84285714 0.85714286 0.87142857 0.88571429 0.9 0.91428571 0.92857143 0.94285714 0.95714286 0.97142857 0.98571429 1 1 1 1 1 1
  arc A18 (-3.4353, -63.407) -> (3.4353, -63.407) centre (0, 0) ccw
  spline S9 degree 5 poles (10.0097, -46.6751) (10.0198, -46.7226) (10.0383, -46.8178) (10.0605, -46.9612) (10.0796, -47.1537) (10.0893, -47.3962) (10.0891, -47.6398) (10.0829, -47.8842) (10.0736, -48.129) (10.0619, -48.374) (10.0476, -48.6191) (10.0296, -48.8645) (10.007, -49.1102) (9.9792, -49.3562) (9.9463, -49.6025) (9.9089, -49.849) (9.8676, -50.0955) (9.8231, -50.3422) (9.7758, -50.5887) (9.7255, -50.8353) (9.6724, -51.0817) (9.6161, -51.3281) (9.5567, -51.5744) (9.4939, -51.8206) (9.428, -52.0667) (9.3591, -52.3127) (9.2873, -52.5584) (9.2128, -52.804) (9.1355, -53.0494) (9.0557, -53.2944) (8.9732, -53.5393) (8.8881, -53.7839) (8.8003, -54.0281) (8.71, -54.2721) (8.617, -54.5158) (8.5215, -54.7591) (8.4236, -55.0021) (8.3232, -55.2447) (8.2204, -55.487) (8.1152, -55.7288) (8.0077, -55.9702) (7.8978, -56.2112) (7.7856, -56.4518) (7.6711, -56.6919) (7.5543, -56.9315) (7.4353, -57.1707) (7.314, -57.4094) (7.1905, -57.6476) (7.0648, -57.8853) (6.937, -58.1224) (6.807, -58.3591) (6.6749, -58.5951) (6.5406, -58.8307) (6.4043, -59.0656) (6.2659, -59.3) (6.1254, -59.5337) (5.9828, -59.7669) (5.8383, -59.9994) (5.6917, -60.2314) (5.5431, -60.4627) (5.3925, -60.6933) (5.24, -60.9233) (5.0855, -61.1526) (4.929, -61.3813) (4.7706, -61.6093) (4.6103, -61.8365) (4.4481, -62.0631) (4.2841, -62.2889) (4.1181, -62.5141) (3.9503, -62.7384) (3.7806, -62.9621) (3.6434, -63.1404) (3.5397, -63.2738) (3.4702, -63.3626) (3.4353, -63.407) knots 0 0 0 0 0 0 0.01428571 0.02857143 0.04285714 0.05714286 0.07142857 0.08571429 0.1 0.11428571 0.12857143 0.14285714 0.15714286 0.17142857 0.18571429 0.2 0.21428571 0.22857143 0.24285714 0.25714286 0.27142857 0.28571429 0.3 0.31428571 0.32857143 0.34285714 0.35714286 0.37142857 0.38571429 0.4 0.41428571 0.42857143 0.44285714 0.45714286 0.47142857 0.48571429 0.5 0.51428571 0.52857143 0.54285714 0.55714286 0.57142857 0.58571429 0.6 0.61428571 0.62857143 0.64285714 0.65714286 0.67142857 0.68571429 0.7 0.71428571 0.72857143 0.74285714 0.75714286 0.77142857 0.78571429 0.8 0.81428571 0.82857143 0.84285714 0.85714286 0.87142857 0.88571429 0.9 0.91428571 0.92857143 0.94285714 0.95714286 0.97142857 0.98571429 1 1 1 1 1 1
  line L9 (10.0097, -46.6751) -> (7.7732, -36.2381)
  arc A19 (8.9264, -34.3689) -> (7.7732, -36.2381) centre (9.3255, -35.9054) ccw
  arc A20 (8.9264, -34.3689) -> (17.9906, -30.6144) centre (0, 0) ccw
  arc A21 (20.1277, -31.1207) -> (17.9906, -30.6144) centre (18.7949, -31.9831) ccw
  line L10 (20.1277, -31.1207) -> (25.9264, -40.0822)
  spline S10 degree 5 poles (25.9264, -40.0822) (25.9528, -40.123) (26.007, -40.2033) (26.0927, -40.3204) (26.2154, -40.4701) (26.3799, -40.6484) (26.5524, -40.8205) (26.7296, -40.989) (26.9092, -41.1554) (27.0907, -41.3204) (27.2742, -41.4836) (27.4604, -41.6444) (27.6501, -41.8022) (27.8437, -41.9565) (28.0411, -42.1074) (28.2419, -42.2552) (28.4454, -42.4004) (28.6513, -42.5433) (28.8591, -42.6841) (29.069, -42.823) (29.2808, -42.9596) (29.4948, -43.0941) (29.711, -43.2262) (29.9295, -43.3559) (30.1501, -43.4833) (30.3728, -43.6085) (30.5973, -43.7315) (30.8237, -43.8525) (31.0517, -43.9714) (31.2815, -44.0882) (31.513, -44.203) (31.7461, -44.3158) (31.9809, -44.4264) (32.2173, -44.5351) (32.4553, -44.6416) (32.6949, -44.7462) (32.936, -44.8487) (33.1785, -44.9493) (33.4225, -45.0479) (33.6679, -45.1445) (33.9146, -45.2392) (34.1627, -45.3319) (34.4122, -45.4227) (34.6629, -45.5115) (34.915, -45.5984) (35.1683, -45.6833) (35.4228, -45.7664) (35.6786, -45.8475) (35.9355, -45.9267) (36.1936, -46.004) (36.4528, -46.0794) (36.7132, -46.1529) (36.9746, -46.2245) (37.2372, -46.2942) (37.5008, -46.362) (37.7654, -46.428) (38.0311, -46.4921) (38.2977, -46.5543) (38.5654, -46.6146) (38.834, -46.6731) (39.1036, -46.7297) (39.3741, -46.7845) (39.6455, -46.8374) (39.9178, -46.8885) (40.191, -46.9377) (40.465, -46.985) (40.7399, -47.0305) (41.0156, -47.0742) (41.2922, -47.1161) (41.5695, -47.1561) (41.8476, -47.1942) (42.0707, -47.2233) (42.2384, -47.2443) (42.3504, -47.2579) (42.4064, -47.2647) knots 0 0 0 0 0 0 0.01428571 0.02857143 0.04285714 0.05714286 0.07142857 0.08571429 0.1 0.11428571 0.12857143 0.14285714 0.15714286 0.17142857 0.18571429 0.2 0.21428571 0.22857143 0.24285714 0.25714286 0.27142857 0.28571429 0.3 0.31428571 0.32857143 0.34285714 0.35714286 0.37142857 0.38571429 0.4 0.41428571 0.42857143 0.44285714 0.45714286 0.47142857 0.48571429 0.5 0.51428571 0.52857143 0.54285714 0.55714286 0.57142857 0.58571429 0.6 0.61428571 0.62857143 0.64285714 0.65714286 0.67142857 0.68571429 0.7 0.71428571 0.72857143 0.74285714 0.75714286 0.77142857 0.78571429 0.8 0.81428571 0.82857143 0.84285714 0.85714286 0.87142857 0.88571429 0.9 0.91428571 0.92857143 0.94285714 0.95714286 0.97142857 0.98571429 1 1 1 1 1 1
  arc A22 (42.4064, -47.2647) -> (47.2647, -42.4064) centre (0, 0) ccw
  spline S11 degree 5 poles (40.0822, -25.9264) (40.123, -25.9528) (40.2033, -26.007) (40.3204, -26.0927) (40.4701, -26.2154) (40.6484, -26.3799) (40.8205, -26.5524) (40.989, -26.7296) (41.1554, -26.9092) (41.3204, -27.0907) (41.4836, -27.2742) (41.6444, -27.4604) (41.8022, -27.6501) (41.9565, -27.8437) (42.1074, -28.0411) (42.2552, -28.2419) (42.4004, -28.4454) (42.5433, -28.6513) (42.6841, -28.8591) (42.823, -29.069) (42.9596, -29.2808) (43.0941, -29.4948) (43.2262, -29.711) (43.3559, -29.9295) (43.4833, -30.1501) (43.6085, -30.3728) (43.7315, -30.5973) (43.8525, -30.8237) (43.9714, -31.0517) (44.0882, -31.2815) (44.203, -31.513) (44.3158, -31.7461) (44.4264, -31.9809) (44.5351, -32.2173) (44.6416, -32.4553) (44.7462, -32.6949) (44.8487, -32.936) (44.9493, -33.1785) (45.0479, -33.4225) (45.1445, -33.6679) (45.2392, -33.9146) (45.3319, -34.1627) (45.4227, -34.4122) (45.5115, -34.6629) (45.5984, -34.915) (45.6833, -35.1683) (45.7664, -35.4228) (45.8475, -35.6786) (45.9267, -35.9355) (46.004, -36.1936) (46.0794, -36.4528) (46.1529, -36.7132) (46.2245, -36.9746) (46.2942, -37.2372) (46.362, -37.5008) (46.428, -37.7654) (46.4921, -38.0311) (46.5543, -38.2977) (46.6146, -38.5654) (46.6731, -38.834) (46.7297, -39.1036) (46.7845, -39.3741) (46.8374, -39.6455) (46.8885, -39.9178) (46.9377, -40.191) (46.985, -40.465) (47.0305, -40.7399) (47.0742, -41.0156) (47.1161, -41.2922) (47.1561, -41.5695) (47.1942, -41.8476) (47.2233, -42.0707) (47.2443, -42.2384) (47.2579, -42.3504) (47.2647, -42.4064) knots 0 0 0 0 0 0 0.01428571 0.02857143 0.04285714 0.05714286 0.07142857 0.08571429 0.1 0.11428571 0.12857143 0.14285714 0.15714286 0.17142857 0.18571429 0.2 0.21428571 0.22857143 0.24285714 0.25714286 0.27142857 0.28571429 0.3 0.31428571 0.32857143 0.34285714 0.35714286 0.37142857 0.38571429 0.4 0.41428571 0.42857143 0.44285714 0.45714286 0.47142857 0.48571429 0.5 0.51428571 0.52857143 0.54285714 0.55714286 0.57142857 0.58571429 0.6 0.61428571 0.62857143 0.64285714 0.65714286 0.67142857 0.68571429 0.7 0.71428571 0.72857143 0.74285714 0.75714286 0.77142857 0.78571429 0.8 0.81428571 0.82857143 0.84285714 0.85714286 0.87142857 0.88571429 0.9 0.91428571 0.92857143 0.94285714 0.95714286 0.97142857 0.98571429 1 1 1 1 1 1
  line L11 (40.0822, -25.9264) -> (31.1207, -20.1277)
  arc A23 (30.6144, -17.9906) -> (31.1207, -20.1277) centre (31.9831, -18.7949) ccw
  arc A24 (30.6144, -17.9906) -> (34.3689, -8.9264) centre (0, 0) ccw
  arc A25 (36.2381, -7.7732) -> (34.3689, -8.9264) centre (35.9054, -9.3255) ccw
  line L12 (36.2381, -7.7732) -> (46.6751, -10.0097)
  spline S12 degree 5 poles (46.6751, -10.0097) (46.7226, -10.0198) (46.8178, -10.0383) (46.9612, -10.0605) (47.1537, -10.0796) (47.3962, -10.0893) (47.6398, -10.0891) (47.8842, -10.0829) (48.129, -10.0736) (48.374, -10.0619) (48.6191, -10.0476) (48.8645, -10.0296) (49.1102, -10.007) (49.3562, -9.9792) (49.6025, -9.9463) (49.849, -9.9089) (50.0955, -9.8676) (50.3422, -9.8231) (50.5887, -9.7758) (50.8353, -9.7255) (51.0817, -9.6724) (51.3281, -9.6161) (51.5744, -9.5567) (51.8206, -9.4939) (52.0667, -9.428) (52.3127, -9.3591) (52.5584, -9.2873) (52.804, -9.2128) (53.0494, -9.1355) (53.2944, -9.0557) (53.5393, -8.9732) (53.7839, -8.8881) (54.0281, -8.8003) (54.2721, -8.71) (54.5158, -8.617) (54.7591, -8.5215) (55.0021, -8.4236) (55.2447, -8.3232) (55.487, -8.2204) (55.7288, -8.1152) (55.9702, -8.0077) (56.2112, -7.8978) (56.4518, -7.7856) (56.6919, -7.6711) (56.9315, -7.5543) (57.1707, -7.4353) (57.4094, -7.314) (57.6476, -7.1905) (57.8853, -7.0648) (58.1224, -6.937) (58.3591, -6.807) (58.5951, -6.6749) (58.8307, -6.5406) (59.0656, -6.4043) (59.3, -6.2659) (59.5337, -6.1254) (59.7669, -5.9828) (59.9994, -5.8383) (60.2314, -5.6917) (60.4627, -5.5431) (60.6933, -5.3925) (60.9233, -5.24) (61.1526, -5.0855) (61.3813, -4.929) (61.6093, -4.7706) (61.8365, -4.6103) (62.0631, -4.4481) (62.2889, -4.2841) (62.5141, -4.1181) (62.7384, -3.9503) (62.9621, -3.7806) (63.1404, -3.6434) (63.2738, -3.5397) (63.3626, -3.4702) (63.407, -3.4353) knots 0 0 0 0 0 0 0.01428571 0.02857143 0.04285714 0.05714286 0.07142857 0.08571429 0.1 0.11428571 0.12857143 0.14285714 0.15714286 0.17142857 0.18571429 0.2 0.21428571 0.22857143 0.24285714 0.25714286 0.27142857 0.28571429 0.3 0.31428571 0.32857143 0.34285714 0.35714286 0.37142857 0.38571429 0.4 0.41428571 0.42857143 0.44285714 0.45714286 0.47142857 0.48571429 0.5 0.51428571 0.52857143 0.54285714 0.55714286 0.57142857 0.58571429 0.6 0.61428571 0.62857143 0.64285714 0.65714286 0.67142857 0.68571429 0.7 0.71428571 0.72857143 0.74285714 0.75714286 0.77142857 0.78571429 0.8 0.81428571 0.82857143 0.84285714 0.85714286 0.87142857 0.88571429 0.9 0.91428571 0.92857143 0.94285714 0.95714286 0.97142857 0.98571429 1 1 1 1 1 1
  arc A26 (63.407, -3.4353) -> (63.407, 3.4353) centre (0, 0) ccw
  spline S13 degree 5 poles (46.6751, 10.0097) (46.7226, 10.0198) (46.8178, 10.0383) (46.9612, 10.0605) (47.1537, 10.0796) (47.3962, 10.0893) (47.6398, 10.0891) (47.8842, 10.0829) (48.129, 10.0736) (48.374, 10.0619) (48.6191, 10.0476) (48.8645, 10.0296) (49.1102, 10.007) (49.3562, 9.9792) (49.6025, 9.9463) (49.849, 9.9089) (50.0955, 9.8676) (50.3422, 9.8231) (50.5887, 9.7758) (50.8353, 9.7255) (51.0817, 9.6724) (51.3281, 9.6161) (51.5744, 9.5567) (51.8206, 9.4939) (52.0667, 9.428) (52.3127, 9.3591) (52.5584, 9.2873) (52.804, 9.2128) (53.0494, 9.1355) (53.2944, 9.0557) (53.5393, 8.9732) (53.7839, 8.8881) (54.0281, 8.8003) (54.2721, 8.71) (54.5158, 8.617) (54.7591, 8.5215) (55.0021, 8.4236) (55.2447, 8.3232) (55.487, 8.2204) (55.7288, 8.1152) (55.9702, 8.0077) (56.2112, 7.8978) (56.4518, 7.7856) (56.6919, 7.6711) (56.9315, 7.5543) (57.1707, 7.4353) (57.4094, 7.314) (57.6476, 7.1905) (57.8853, 7.0648) (58.1224, 6.937) (58.3591, 6.807) (58.5951, 6.6749) (58.8307, 6.5406) (59.0656, 6.4043) (59.3, 6.2659) (59.5337, 6.1254) (59.7669, 5.9828) (59.9994, 5.8383) (60.2314, 5.6917) (60.4627, 5.5431) (60.6933, 5.3925) (60.9233, 5.24) (61.1526, 5.0855) (61.3813, 4.929) (61.6093, 4.7706) (61.8365, 4.6103) (62.0631, 4.4481) (62.2889, 4.2841) (62.5141, 4.1181) (62.7384, 3.9503) (62.9621, 3.7806) (63.1404, 3.6434) (63.2738, 3.5397) (63.3626, 3.4702) (63.407, 3.4353) knots 0 0 0 0 0 0 0.01428571 0.02857143 0.04285714 0.05714286 0.07142857 0.08571429 0.1 0.11428571 0.12857143 0.14285714 0.15714286 0.17142857 0.18571429 0.2 0.21428571 0.22857143 0.24285714 0.25714286 0.27142857 0.28571429 0.3 0.31428571 0.32857143 0.34285714 0.35714286 0.37142857 0.38571429 0.4 0.41428571 0.42857143 0.44285714 0.45714286 0.47142857 0.48571429 0.5 0.51428571 0.52857143 0.54285714 0.55714286 0.57142857 0.58571429 0.6 0.61428571 0.62857143 0.64285714 0.65714286 0.67142857 0.68571429 0.7 0.71428571 0.72857143 0.74285714 0.75714286 0.77142857 0.78571429 0.8 0.81428571 0.82857143 0.84285714 0.85714286 0.87142857 0.88571429 0.9 0.91428571 0.92857143 0.94285714 0.95714286 0.97142857 0.98571429 1 1 1 1 1 1
  line L13 (46.6751, 10.0097) -> (36.2381, 7.7732)
  arc A27 (34.3689, 8.9264) -> (36.2381, 7.7732) centre (35.9054, 9.3255) ccw
  arc A28 (34.3689, 8.9264) -> (30.6144, 17.9906) centre (0, 0) ccw
  arc A29 (31.1207, 20.1277) -> (30.6144, 17.9906) centre (31.9831, 18.7949) ccw
  line L14 (31.1207, 20.1277) -> (40.0822, 25.9264)
  spline S14 degree 5 poles (40.0822, 25.9264) (40.123, 25.9528) (40.2033, 26.007) (40.3204, 26.0927) (40.4701, 26.2154) (40.6484, 26.3799) (40.8205, 26.5524) (40.989, 26.7296) (41.1554, 26.9092) (41.3204, 27.0907) (41.4836, 27.2742) (41.6444, 27.4604) (41.8022, 27.6501) (41.9565, 27.8437) (42.1074, 28.0411) (42.2552, 28.2419) (42.4004, 28.4454) (42.5433, 28.6513) (42.6841, 28.8591) (42.823, 29.069) (42.9596, 29.2808) (43.0941, 29.4948) (43.2262, 29.711) (43.3559, 29.9295) (43.4833, 30.1501) (43.6085, 30.3728) (43.7315, 30.5973) (43.8525, 30.8237) (43.9714, 31.0517) (44.0882, 31.2815) (44.203, 31.513) (44.3158, 31.7461) (44.4264, 31.9809) (44.5351, 32.2173) (44.6416, 32.4553) (44.7462, 32.6949) (44.8487, 32.936) (44.9493, 33.1785) (45.0479, 33.4225) (45.1445, 33.6679) (45.2392, 33.9146) (45.3319, 34.1627) (45.4227, 34.4122) (45.5115, 34.6629) (45.5984, 34.915) (45.6833, 35.1683) (45.7664, 35.4228) (45.8475, 35.6786) (45.9267, 35.9355) (46.004, 36.1936) (46.0794, 36.4528) (46.1529, 36.7132) (46.2245, 36.9746) (46.2942, 37.2372) (46.362, 37.5008) (46.428, 37.7654) (46.4921, 38.0311) (46.5543, 38.2977) (46.6146, 38.5654) (46.6731, 38.834) (46.7297, 39.1036) (46.7845, 39.3741) (46.8374, 39.6455) (46.8885, 39.9178) (46.9377, 40.191) (46.985, 40.465) (47.0305, 40.7399) (47.0742, 41.0156) (47.1161, 41.2922) (47.1561, 41.5695) (47.1942, 41.8476) (47.2233, 42.0707) (47.2443, 42.2384) (47.2579, 42.3504) (47.2647, 42.4064) knots 0 0 0 0 0 0 0.01428571 0.02857143 0.04285714 0.05714286 0.07142857 0.08571429 0.1 0.11428571 0.12857143 0.14285714 0.15714286 0.17142857 0.18571429 0.2 0.21428571 0.22857143 0.24285714 0.25714286 0.27142857 0.28571429 0.3 0.31428571 0.32857143 0.34285714 0.35714286 0.37142857 0.38571429 0.4 0.41428571 0.42857143 0.44285714 0.45714286 0.47142857 0.48571429 0.5 0.51428571 0.52857143 0.54285714 0.55714286 0.57142857 0.58571429 0.6 0.61428571 0.62857143 0.64285714 0.65714286 0.67142857 0.68571429 0.7 0.71428571 0.72857143 0.74285714 0.75714286 0.77142857 0.78571429 0.8 0.81428571 0.82857143 0.84285714 0.85714286 0.87142857 0.88571429 0.9 0.91428571 0.92857143 0.94285714 0.95714286 0.97142857 0.98571429 1 1 1 1 1 1
  arc A30 (47.2647, 42.4064) -> (42.4064, 47.2647) centre (0, 0) ccw